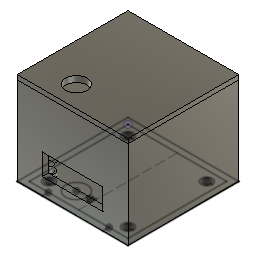
Single PWM Fan Controller (Autodesk Fusion 360 design; units mm, degrees)
Autodesk Fusion 360 part; units mm, degrees
sketch "Bottom" plane through (0, 0, 0) normal (0, 0, 1) x (1, 0, 0) in component "Case"
  line L0 (0, 0) -> (32.5, 0)
  line L1 (32.5, 0) -> (32.5, -32.5)
  line L2 (32.5, -32.5) -> (0, -32.5)
  line L3 (0, -32.5) -> (0, 0)
  line L4 (34.5, -34.5) -> (-2, -34.5)
  line L5 (-2, -34.5) -> (-2, 2)
  line L6 (-2, 2) -> (34.5, 2)
  line L7 (34.5, 2) -> (34.5, -34.5)
  circle A0 centre (3.25, -3.25) radius 1.75
  line L8 (16.25, 0) -> (16.25, -32.5) construction
  line L9 (6.25, -32.5) -> (6.25, -34.5)
  line L10 (26.25, -32.5) -> (26.25, -34.5)
  circle A1 centre (10.5, -27.5) radius 3.5
  line L11 (15, -26.5) -> (16, -26.5)
  line L12 (16, -26.5) -> (16, -28.5)
  line L13 (16, -28.5) -> (15, -28.5)
  line L14 (15, -28.5) -> (15, -26.5)
  line L15 (10.5, -27.5) -> (15, -27.5) construction
  circle A2 centre (3.25, -3.25) radius 1.25
  circle A3 centre (29.25, -3.25) radius 1.25
  circle A4 centre (3.25, -29.25) radius 1.25
  circle A5 centre (29.25, -29.25) radius 1.25
  circle A6 centre (29.25, -3.25) radius 1.75
  circle A7 centre (3.25, -29.25) radius 1.75
  circle A8 centre (29.25, -29.25) radius 1.75
  point P0 (6.25, -32.5)
  point P1 (26.25, -32.5)
  point P2 (15, -27.5)
  dimension "d1" = 32.5
  dimension "d2" = 32.5
  dimension "d4" = -2
  dimension "d7" = 3.5
  dimension "d8" = 3.25
  dimension "d9" = 3.25
  dimension "d18" = 20
  dimension "d19" = 10
  dimension "d23" = 7
  dimension "d24" = 5
  dimension "d25" = 10.5
  dimension "d26" = 1
  dimension "d27" = 2
  dimension "d34" = 2.5
  dimension "d37" = 26
  dimension "d38" = -26
  dimension "d39" = 3.75
  dimension "d42" = 4.5
  constraint horizontal L0
  constraint vertical L1
  constraint horizontal L2
  constraint vertical L3
  constraint coincident L0.start L3.end
  constraint midpoint L0 L8.start
  constraint midpoint L2 L8.end
  constraint coincident L2 P0
  constraint coincident L2 P1
  constraint coincident P0 L9.start
  constraint coincident L4 L9.end
  constraint perpendicular L4 L9
  constraint coincident P1 L10.start
  constraint coincident L4 L10.end
  constraint perpendicular L4 L10
  constraint horizontal L11
  constraint vertical L12
  constraint horizontal L13
  constraint vertical L14
  constraint midpoint L14 P2
  constraint coincident A1.centre L15.start
  constraint coincident P2 L15.end
  constraint perpendicular L14 L15
  constraint concentric A0 A2
  measures "d1" distance of L0.start L0.end
  measures "d2" distance of L0.start L2.end
  measures "d7" diameter of A0
  measures "d8" distance of L3 A0.centre
  measures "d9" distance of L0 A0.centre
  measures "d18" distance of P0 P1
  measures "d19" distance of L8.end P0
  measures "d23" diameter of A1
  measures "d24" distance of L2 A1.centre
  measures "d25" distance of L3 A1.centre
  measures "d26" distance of L11.start L11.end
  measures "d27" distance of L11.start L13.end
  measures "d34" diameter of A2
  measures "d42" distance of A1.centre P2
extrude "Extrude1" add sketch "Bottom" along normal blind 1 contours L0 L1 L2 L3 | A0 | A1 | L11 L12 L13 L14 | A2 | A3 | A4 | A5 | A6 | A7 | A8 makes body 1 in component "Case"
extrude "Extrude7" add sketch "Bottom" along normal blind 5 contours A2 | A3 | A4 | A5 bodies 1 in component "Case"
extrude "Extrude2" add sketch "Bottom" along normal blind 3 contours A0 | A2 | A3 | A4 | A5 | A6 | A7 | A8 bodies 1 in component "Case"
extrude "Extrude3" add sketch "Bottom" along normal blind 29 contours L0 L1 L2 L3 L4 L5 L6 L7 L9 L10 | L2 L4 L9 L10 bodies 1 in component "Case"
extrude "Extrude4" cut sketch "Bottom" along normal blind 7 from surface at 5.5 contours L2 L4 L9 L10 bodies 1 in component "Case"
sketch "Sketch3" plane through (0, 0, 29) normal (0, 0, 1) x (-1, 0, 0) in component "Case"
  line L0 (-32.5, 32.5) -> (0, 32.5)
  line L1 (0, 32.5) -> (0, 0)
  line L2 (0, 0) -> (-32.5, 0)
  line L3 (-32.5, 0) -> (-32.5, 32.5)
  line L4 (-34.5, -2) -> (2, -2)
  line L5 (2, -2) -> (2, 34.5)
  line L6 (2, 34.5) -> (-34.5, 34.5)
  line L7 (-34.5, 34.5) -> (-34.5, -2)
  line L8 (0, 32.5) -> (0, 0)
  line L9 (-32.5, 32.5) -> (0, 32.5)
  circle A0 centre (-10.5, 27.5) radius 3.5
  line L10 (-16, 28.5) -> (-15, 28.5)
  line L11 (-16, 26.5) -> (-16, 28.5)
  line L12 (-15, 26.5) -> (-16, 26.5)
  line L13 (-15, 28.5) -> (-15, 26.5)
  line L14 (-32.5, 0) -> (-32.5, 32.5)
  line L15 (0, 0) -> (-32.5, 0)
  line L16 (-0.1, 32.4) -> (-0.1, 0.1)
  line L17 (-0.1, 0.1) -> (-32.4, 0.1)
  line L18 (-32.4, 0.1) -> (-32.4, 32.4)
  line L19 (-32.4, 32.4) -> (-0.1, 32.4)
  line L20 (2, -2) -> (-34.5, -2)
  line L21 (-34.5, 34.5) -> (-34.5, -2)
  line L22 (2, 34.5) -> (-34.5, 34.5)
  line L23 (2, 34.5) -> (2, -2)
  circle A1 centre (-10.5, 27.5) radius 3.5
  circle A2 centre (-10.5, 27.5) radius 3.5
  line L24 (-15, 26.5) -> (-16, 26.5)
  line L25 (-16, 28.5) -> (-15, 28.5)
  point P0 (-15, 28.5)
  dimension "d29" = 0.1
  constraint coincident L4.end L5.start
  constraint coincident L4.start L7.end
  constraint coincident L6.end L7.start
  constraint coincident L5.end L6.start
  constraint perpendicular L5 L22
  constraint concentric A0 A1
  constraint concentric A1 A2
  constraint coincident L12.start L13.end
  constraint coincident L11.start L12.end
  constraint coincident L10.start L11.end
  constraint coincident P0 L10.end
extrude "Extrude5" add sketch "Sketch3" against normal blind 0.5 separate body contours L16 L17 L18 L19 makes body 2 in component "Case"
extrude "Extrude6" add sketch "Sketch3" along normal blind 1.5 contours L0 L1 L2 L3 L8 L9 L14 L15 | L4 L5 L6 L7 L20 L21 L22 L23 | L10 L11 L12 L13 L24 L25 | L16 L17 L18 L19 bodies 2 in component "Case"
component "Case" placed x (1, 0, 0) y (0, 1, 0) z (0, 0, 1) at (0, 0, 0)
named bodies: "Bottom", "Top"
